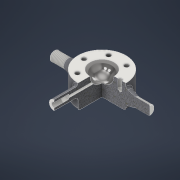
# Autodesk Inventor part: Деталь1
Saved by Autodesk Inventor 2022 (Build 260153000, 153)
## iProperties
Created: 2023-04-26
Part Number: Деталь1
Material: Чугун, литейный
Document SubType Name: Modeling
Designer: lxve_every1
Density: 7.15 g/cm^3
Appearance: Сталь
Author: lxve_every1
Autodesk Inventor part; units mm, degrees
ref_plane "XZ Plane" through (0, 0, 0) normal (0, 1, 0) x (-1, 0, 0)
ref_plane "XY Plane" through (0, 0, 0) normal (0, 0, 1) x (1, 0, 0)
ref_plane "РабПлоскость1" through (0, 0, 25) normal (0, 0, 1) x (1, 0, 0)
sketch "Эскиз5" plane through (0, 0, 0) normal (0, 0, 1) x (1, 0, 0)
  circle A0 centre (0, 0) radius 50
  dimension "d4" = 100
  constraints: 1 centre point, 1 coincident
  measures "d4" diameter of A0
extrude "Выдавливание" add sketch "Эскиз5" along normal blind 50
sketch "Эскиз6" plane through (0, 0, 25) normal (0, 0, 1) x (1, 0, 0)
  line L0 (0, -14.0192) -> (0, -100)
  line L1 (0, -100) -> (-10, -100)
  line L2 (-10, -100) -> (-10, -70)
  line L3 (-10, -70) -> (-25, -14.0192)
  line L4 (-25, -14.0192) -> (0, -14.0192)
  point P0 (0, 0)
  dimension "d7" = 100
  dimension "d8" = 10
  dimension "d9" = 30
  dimension "d10" = 25
  dimension "d11" = 15
  constraints: 10 end point, 3 perpendicular
  measures "d7" distance of point (0, 0) L0.end
  measures "d8" distance of L0.end L1.end
  measures "d9" distance of L1.end L2.end
  measures "d10" distance of L0.start L3.end
  measures "d11" angle of L3 L2
revolve "Вращение1" add sketch "Эскиз6" angle 360 about axis through (0, -14.0192, 25) along (0, -1, 0)
thread "Резьба1" size "M20x2.5" class "6g" standard "ISO Metric profile" full length
chamfer "Фаска1" distance 1.6 angle 45 1 edges at (10, -100, 25)
fillet "Сопряжение1" radius 5 1 edges at (16.0698, -47.3472, 24.9987)
mirror "Зеркальное отражение1" about plane through (0, 0, 0) normal (0, 1, 0) of "Вращение1", "Фаска1", "Сопряжение1"
ref_plane "РабПлоскость3" through (50, 0, 0) normal (1, 0, 0) x (0, 1, 0)
sketch "Эскиз9" plane through (50, 0, 0) normal (1, 0, 0) x (0, 1, 0)
  line L0 (0, 0) -> (0, 35)
  circle A0 centre (0, 35) radius 10
  dimension "d22" = 35
  dimension "d23" = 20
  constraints: 2 end point, 1 centre point, 1 coincident, 1 vertical
  measures "d22" distance of L0.start L0.end
  measures "d23" diameter of A0
extrude "Выдавливание2" add sketch "Эскиз9" along normal blind 50 and the other way blind 15.25
fillet "Сопряжение2" radius 5 3 edges at (48.9898, -10, 35.0018) (49.4151, 7.6255, 41.4693) (49.4151, 7.6255, 28.5307)
fillet "Сопряжение3" radius 5 1 edges at (-50, 0, 0)
sketch "Эскиз10" plane through (0, 0, 50) normal (0, 0, 1) x (1, 0, 0)
  circle A0 centre (0, 0) radius 45 projected
  arc A1 (-25, 0) -> (25, 0) centre (0, 0) ccw
  line L0 (25, 0) -> (-25, 0)
  arc A2 (25, 0) -> (-25, 0) centre (0, 0) ccw
  dimension "d30" = 50
  constraints: 4 point on circle, 2 centre point, 2 end point, 1 coincident, 1 horizontal, 1 other
  measures "d30" diameter of A1
revolve "Вращение2" cut sketch "Эскиз10" angle 360 about axis through (25, 0, 50) along (-1, 0, 0) contours L0 A1
sketch "Эскиз15" plane through (100, 0, 35) normal (1, 0, 0) x (0, 0, -1)
  circle A0 centre (0, 0) radius 6
  point P0 (35, 0)
  dimension "d33" = 12
  constraints: 1 centre point
  measures "d33" diameter of A0
hole "Отверстие1" at (100, 0, 35) direction (-1, 0, 0) diameter 10.106 depth 30 tip angle 120 countersink diameter 12 countersink angle 120 thread size "M12x1.75" class "6H" standard "ISO Metric profile"
sketch "Эскиз16" plane through (0, 0, 50) normal (0, 0, 1) x (1, 0, 0)
  line L0 (0, 0) -> (0, -50)
  circle A0 centre (0, 0) radius 50 projected
  line L1 (0, 0) -> (61.1717, -35.3175)
  point P0 (32.476, -18.75)
  dimension "d57" = 60
  constraints: 4 end point, 1 coincident, 1 point on line, 1 vertical, 1 vertical alignment, 1 other
  measures "d57" angle of L1 L0
hole "Отверстие2" at (32.476, -18.75, 50) direction (0, 0, -1) diameter 8.376 depth 20 tip angle 120 countersink diameter 10 countersink angle 120 thread size "M10x1.5" class "6H" standard "ISO Metric profile"
pattern_circular "Круговой массив1" count 6 over 360 about axis through (0, 0, 0) along (0, 0, 1) of "Отверстие2"
sketch "Эскиз17" plane through (100, 0, 35) normal (1, 0, 0) x (0, 0, -1)
  circle A0 centre (0, 0) radius 2.5
  point P0 (35, 0)
  dimension "d54" = 5
  constraints: 1 centre point
  measures "d54" diameter of A0
extrude "Выдавливание3" cut sketch "Эскиз17" against normal up to surface
